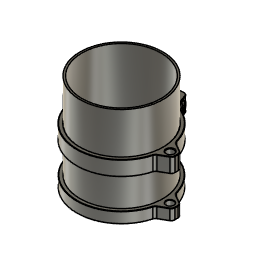
rear_44mm (Autodesk Fusion 360 design; units mm, degrees)
Autodesk Fusion 360 part; units mm, degrees
sketch "Sketch1" plane through (0, 0, 0) normal (0, 0, 1) x (1, 0, 0)
  circle A0 centre (0, 0) radius 22.2
  circle A1 centre (0, 0) radius 21.2
  dimension "d1" = 44.4
  dimension "d2" = 1
  constraint coincident A0.centre A1.centre
  measures "d1" diameter of A0
  measures "d2" distance of A0 A1
extrude "Extrude1" add sketch "Sketch1" along normal blind 50 makes body 1
ref_plane "WorkPlane1" through (0, 0, 20) normal (0, 0, 1) x (1, 0, 0)
sketch "Sketch2" plane through (0, 0, 20) normal (0, 0, 1) x (1, 0, 0)
  circle A0 centre (0, 0) radius 22.1
  circle A1 centre (0, 0) radius 24.1
  line L0 (0, 0) -> (0, 24.1) construction
  line L1 (-6.9118, 23.0876) -> (-4, 31.0876)
  line L2 (-4, 31.0876) -> (0, 31.0876)
  line L3 (0, 31.0876) -> (0, 24.1)
  line L4 (-6.9118, 23.0876) -> (0, 23.0876) construction
  line L5 (-4, 31.0876) -> (-4, 23.0876) construction
  line L6 (0, 0) -> (-0.3086, 22.0978)
  line L7 (-0.3086, 22.0978) -> (-0.3086, 31.0876)
  line L8 (6.9118, 23.0876) -> (4, 31.0876)
  line L9 (4, 31.0876) -> (0, 31.0876)
  line L10 (0.3086, 22.0978) -> (0.3086, 31.0876)
  line L11 (0, 0) -> (0.3086, 22.0978)
  circle A2 centre (-26.1, 0) radius 2
  line L12 (0, 0) -> (-24.1, 0) construction
  line L13 (-23.4467, 5.5733) -> (-29.6, 2.0207)
  line L14 (-29.6, 2.0207) -> (-29.6, 0)
  line L15 (-23.4467, -5.5733) -> (-29.6, -2.0207)
  line L16 (-29.6, -2.0207) -> (-29.6, 0)
  line L17 (23.4467, 5.5733) -> (29.6, 2.0207)
  line L18 (29.6, 2.0207) -> (29.6, 0)
  line L19 (29.6, -2.0207) -> (29.6, 0)
  line L20 (23.4467, -5.5733) -> (29.6, -2.0207)
  circle A3 centre (26.1, 0) radius 2
  dimension "d6" = 44.2
  dimension "d7" = 2
  dimension "d8" = 8
  dimension "d9" = 20
  dimension "d10" = 4
  dimension "d11" = 0.8
  dimension "d14" = 4
  dimension "d16" = 3.5
  dimension "d17" = 3.5
  dimension "d18" = 120
  constraint coincident A0.centre A1.centre
  constraint coincident A1 L0.end
  constraint vertical L0
  constraint coincident A1 L1.start
  constraint horizontal L2
  constraint perpendicular L2 L3
  constraint coincident L0 L4.end
  constraint horizontal L4
  constraint coincident L4 L5.end
  constraint perpendicular L4 L5
  constraint coincident A0 L6.end
  constraint coincident L2 L7.end
  constraint perpendicular L2 L7
  constraint symmetric L0 L1.start L8.start
  constraint symmetric L0 L1.end L8.end
  constraint symmetric L0 L2.end L3.start
  constraint symmetric L0 A0.centre A1.centre
  constraint symmetric L0 L6.end L10.start
  constraint symmetric L0 L7.end L10.end
  constraint coincident A1 L12.end
  constraint horizontal L12
  constraint coincident A2.centre L12
  constraint coincident A1 L13.start
  constraint vertical L14
  constraint tangent A1 A2
  constraint coincident L12 L14.end
  constraint symmetric L12 L13.start L15.start
  constraint symmetric L12 L13.end L15.end
  constraint symmetric L12 L14.end L16.end
  constraint symmetric L0 A2 A3
  constraint symmetric L0 L13.start L17.start
  constraint symmetric L0 L13.end L17.end
  constraint symmetric L0 L14.end L18.end
  constraint symmetric L0 L15.start L20.start
  constraint symmetric L0 L15.end L19.start
  measures "d6" diameter of A0
  measures "d7" distance of A0 A1
  measures "d8" distance of L2 L4
  measures "d9" angle of L1 L5
  measures "d10" distance of L1.end L3
  measures "d11" angle of L0 L6
  measures "d14" diameter of A2
  measures "d16" distance of A2.centre L14
  measures "d17" distance of A2.centre L13
  measures "d18" angle of L13 L14
extrude "Extrude2" add sketch "Sketch2" along normal blind 8 separate body contours A0 A1 L7 L10 | A1 L8 L9 L10 | A1 L1 L2 L7 | A1 L17 L18 L19 L20 | A1 L13 L14 L15 L16 picked at (22.6631, -1.702) makes body 2
sketch "Sketch3" plane through (-0.3086, 0, 0) normal (1, 0, 0) x (0, 1, 0)
  line L0 (22.0978, 20) -> (31.0876, 20)
  line L1 (31.0876, 20) -> (31.0876, 28)
  line L2 (31.0876, 28) -> (22.0978, 28)
  line L3 (22.0978, 28) -> (22.0978, 20)
  line L4 (22.0978, 24) -> (31.0876, 24) construction
  line L5 (26.5927, 28) -> (26.5927, 20) construction
  circle A0 centre (27.0876, 24) radius 1.4
  dimension "d19" = 2.8
  dimension "d20" = 4
  constraint midpoint L3 L4.start
  constraint midpoint L1 L4.end
  constraint midpoint L2 L5.start
  constraint perpendicular L2 L5
  constraint coincident L4 A0.centre
  measures "d19" diameter of A0
  measures "d20" distance of L1 A0.centre
extrude "Extrude3" cut sketch "Sketch3" along normal through all and the other way through all contours A0 bodies 2
sketch "Sketch4" plane through (0, 0, 28) normal (0, 0, 1) x (-1, 0, 0)
  circle A0 centre (-26.1, 0) radius 2
  circle A1 centre (26.1, 0) radius 2
  arc A2 (23.4467, 5.5733) -> (-23.4467, 5.5733) centre (0, 0) ccw
  line L0 (-23.4467, 5.5733) -> (-29.6, 2.0207)
  line L1 (-29.6, 2.0207) -> (-29.6, -2.0207)
  line L2 (-29.6, -2.0207) -> (-23.4467, -5.5733)
  arc A3 (-23.4467, -5.5733) -> (-6.9118, -23.0876) centre (0, 0) ccw
  line L3 (-6.9118, -23.0876) -> (-4, -31.0876)
  line L4 (-4, -31.0876) -> (-0.3086, -31.0876)
  line L5 (-0.3086, -31.0876) -> (-0.3086, -22.0978)
  arc A4 (0.3086, -22.0978) -> (-0.3086, -22.0978) centre (0, 0) ccw
  line L6 (0.3086, -22.0978) -> (0.3086, -31.0876)
  line L7 (0.3086, -31.0876) -> (4, -31.0876)
  line L8 (4, -31.0876) -> (6.9118, -23.0876)
  arc A5 (6.9118, -23.0876) -> (23.4467, -5.5733) centre (0, 0) ccw
  line L9 (23.4467, -5.5733) -> (29.6, -2.0207)
  line L10 (29.6, -2.0207) -> (29.6, 2.0207)
  line L11 (29.6, 2.0207) -> (23.4467, 5.5733)
  line L12 (-4, -31.0876) -> (-4, -21.735) construction
  constraint coincident L3.end L4.start
  constraint coincident A4 L12.end
  constraint perpendicular L4 L12
sketch "Sketch5" plane through (0, 0, 20) normal (0, 0, -1) x (1, 0, 0)
  circle A0 centre (26.1, 0) radius 2
  circle A1 centre (-26.1, 0) radius 2
  arc A2 (23.4467, 5.5733) -> (-23.4467, 5.5733) centre (0, 0) ccw
  line L0 (-23.4467, 5.5733) -> (-29.6, 2.0207)
  line L1 (-29.6, 2.0207) -> (-29.6, -2.0207)
  line L2 (-29.6, -2.0207) -> (-23.4467, -5.5733)
  arc A3 (-23.4467, -5.5733) -> (-6.9118, -23.0876) centre (0, 0) ccw
  line L3 (-6.9118, -23.0876) -> (-4, -31.0876)
  line L4 (-4, -31.0876) -> (-0.3086, -31.0876)
  line L5 (-0.3086, -31.0876) -> (-0.3086, -22.0978)
  arc A4 (0.3086, -22.0978) -> (-0.3086, -22.0978) centre (0, 0) ccw
  line L6 (0.3086, -22.0978) -> (0.3086, -31.0876)
  line L7 (0.3086, -31.0876) -> (4, -31.0876)
  line L8 (4, -31.0876) -> (6.9118, -23.0876)
  arc A5 (6.9118, -23.0876) -> (23.4467, -5.5733) centre (0, 0) ccw
  line L9 (23.4467, -5.5733) -> (29.6, -2.0207)
  line L10 (29.6, -2.0207) -> (29.6, 2.0207)
  line L11 (29.6, 2.0207) -> (23.4467, 5.5733)
  line L12 (4, -31.0876) -> (4, -21.735) construction
ref_plane "WorkPlane2" through (4, 31.0876, 28) normal (-1, 0, 0) x (0, -1, 0)
sketch "Sketch6" plane through (4, 0, 0) normal (-1, 0, 0) x (0, -1, 0)
  circle A0 centre (-27.0876, 24) radius 1.4
  circle A1 centre (-27.0876, 24) radius 1.4
  circle A2 centre (-27.0876, 24) radius 3
  dimension "d23" = 6
  constraint concentric A0 A2
  measures "d23" diameter of A2
extrude "Extrude4" cut sketch "Sketch6" against normal through all bodies 2
sketch "Sketch7" plane through (0.3086, 0, 0) normal (-1, 0, 0) x (0, -1, 0)
  circle A0 centre (-27.0876, 24) radius 1.4
  line L0 (-31.0876, 20) -> (-22.0978, 20)
  line L1 (-22.0978, 20) -> (-22.0978, 28)
  line L2 (-22.0978, 28) -> (-31.0876, 28)
  line L3 (-31.0876, 28) -> (-31.0876, 20)
  circle A1 centre (-27.0876, 24) radius 1.7
  dimension "d28" = 3.4
  constraint concentric A0 A1
  measures "d28" diameter of A1
extrude "Extrude6" cut sketch "Sketch7" against normal up to surface (3.6914 mm away) contours A1 bodies 2
fillet "Fillet1" radius 2 12 edges at (-29.6, -2.0207, 24) (-23.4467, -5.5733, 24) (-29.6, 2.0207, 24) (-23.4467, 5.5733, 24) (23.4467, -5.5733, 24) (29.6, -2.0207, 24) (29.6, 2.0207, 24) (23.4467, 5.5733, 24) (6.9118, 23.0876, 24) (-6.9118, 23.0876, 24) (4, 31.0876, 24) (-4, 31.0876, 24) on bodies 2
fillet "Fillet2" radius 0.5 4 edges at (0.3086, 31.0876, 24) (-0.3086, 31.0876, 24) (0.3086, 22.0978, 24) (-0.3086, 22.0978, 24) on bodies 2
chamfer "Chamfer1" distance 0.2 angle 45 4 edges at (4, 28.6726, 23.3853) (0.3086, 28.6726, 24.6147) (-0.3086, 25.7823, 24.5063) (-5.9654, 25.6876, 24) on bodies 2
fillet "Fillet5" radius 0.2 3 edges at (4, 29.8846, 22.9152) (6.5478, 24.0876, 24) (4.3316, 30.0876, 24) on bodies 2
chamfer "Chamfer2" distance 0.2 angle 45 32 edges at (-23.5921, 5.6629, 28) (-17.5696, 16.496, 28) (-7.0555, 23.2645, 28) (-5.5278, 26.8899, 28) (-3.7467, 30.7259, 28) (-1.7041, 31.0876, 28) (-0.455, 30.9412, 28) (-0.3086, 26.5866, 28) (-0.4487, 22.2384, 28) (0, -22.1, 28) (0.4487, 22.2384, 28) (0.3086, 26.5866, 28) (0.455, 30.9412, 28) (1.7041, 31.0876, 28) (3.7467, 30.7259, 28) (5.5278, 26.8899, 28) (7.0555, 23.2645, 28) (17.5696, 16.496, 28) (23.5921, 5.6629, 28) (26.3878, 3.8753, 28) (29.3321, 1.866, 28) (29.6, 0, 28) (29.3321, -1.866, 28) (26.3878, -3.8753, 28) (23.5921, -5.6629, 28) (0, -24.1, 28) (-23.5921, -5.6629, 28) (-26.3878, -3.8753, 28) (-29.3321, -1.866, 28) (-29.6, 0, 28) (-29.3321, 1.866, 28) (-26.3878, 3.8753, 28) on bodies 2
chamfer "Chamfer3" distance 0.3 angle 45 36 edges at (-27.9647, 0.7232, 28) (24.2353, 0.7232, 28) (26.3878, 3.8753, 20) (29.3321, 1.866, 20) (29.6, 0, 20) (29.3321, -1.866, 20) (26.3878, -3.8753, 20) (23.5921, -5.6629, 20) (0, -24.1, 20) (-23.5921, -5.6629, 20) (-26.3878, -3.8753, 20) (-29.3321, -1.866, 20) (-29.6, 0, 20) (-29.3321, 1.866, 20) (-26.3878, 3.8753, 20) (-23.5921, 5.6629, 20) (-17.5696, 16.496, 20) (-7.0555, 23.2645, 20) (-5.5278, 26.8899, 20) (-3.7467, 30.7259, 20) (-1.7041, 31.0876, 20) (-0.455, 30.9412, 20) (-0.3086, 26.5866, 20) (-0.4487, 22.2384, 20) (0, -22.1, 20) (0.4487, 22.2384, 20) (0.3086, 26.5866, 20) (0.455, 30.9412, 20) (1.7041, 31.0876, 20) (3.7467, 30.7259, 20) (5.5278, 26.8899, 20) (7.0555, 23.2645, 20) (17.5696, 16.496, 20) (23.5921, 5.6629, 20) (24.2353, 0.7232, 20) (-27.9647, 0.7232, 20) on bodies 2
sketch "Sketch8" plane through (0, 0, 0) normal (0, 0, 1) x (1, 0, 0)
  circle A0 centre (0, 0) radius 22
  circle A1 centre (0, 0) radius 24
  line L0 (23.3435, 5.5752) -> (29.5, 2.0207)
  line L1 (29.5, 2.0207) -> (29.5, 0)
  line L2 (0, 0) -> (24, 0) construction
  line L3 (23.3435, -5.5752) -> (29.5, -2.0207)
  line L4 (29.5, -2.0207) -> (29.5, 0)
  line L5 (0, 0) -> (0, 22) construction
  line L6 (-23.3435, 5.5752) -> (-29.5, 2.0207)
  line L7 (-29.5, 2.0207) -> (-29.5, 0)
  line L8 (-29.5, -2.0207) -> (-29.5, 0)
  line L9 (-23.3435, -5.5752) -> (-29.5, -2.0207)
  circle A2 centre (26, 0) radius 2
  circle A3 centre (-26, 0) radius 2
  line L10 (0, 0) -> (-26, 0) construction
  dimension "d38" = 44
  dimension "d39" = 2
  dimension "d41" = 3.5
  dimension "d42" = 3.5
  dimension "d43" = 120
  dimension "d46" = 4
  dimension "d47" = 4
  constraint coincident A0.centre A1.centre
  constraint coincident A1 L0.start
  constraint vertical L1
  constraint coincident A1 L2.end
  constraint horizontal L2
  constraint symmetric L0.start L2 L3.start
  constraint symmetric L0.end L2 L3.end
  constraint symmetric L1.end L2 L4.end
  constraint coincident A0 L5.end
  constraint perpendicular L2 L5
  constraint symmetric L0.start L5 L6.start
  constraint symmetric L0.end L5 L6.end
  constraint symmetric L1.end L5 L7.end
  constraint symmetric L3.start L5 L9.start
  constraint symmetric L3.end L5 L8.start
  constraint tangent A1 A2
  constraint coincident L2 A2.centre
  constraint tangent A1 A3
  constraint coincident A3.centre L10.end
  constraint horizontal L10
  measures "d38" diameter of A0
  measures "d39" distance of A0 A1
  measures "d41" distance of L0 A2.centre
  measures "d42" distance of L1 A2.centre
  measures "d43" angle of L0 L1
  measures "d46" diameter of A2
  measures "d47" diameter of A3
extrude "Extrude7" add sketch "Sketch8" along normal blind 4 separate body makes body 3
extrude "Extrude8" add sketch "Sketch8" against normal blind 2 contours A0 | A1 | A1 L0 L1 L3 L4 | A1 L6 L7 L8 L9 bodies 3
fillet "Fillet3" radius 2 8 edges at (23.3435, -5.5752, 1) (29.5, -2.0207, 1) (29.5, 2.0207, 1) (23.3435, 5.5752, 1) (-23.3435, 5.5752, 1) (-29.5, 2.0207, 1) (-29.5, -2.0207, 1) (-23.3435, -5.5752, 1) on bodies 3
chamfer "Chamfer4" distance 0.2 angle 45 19 edges at (-29.2321, -1.866, 4) (-29.5, 0, 4) (-29.2321, 1.866, 4) (-26.2856, 3.8765, 4) (-23.4884, 5.6646, 4) (0, 24, 4) (23.4884, 5.6646, 4) (26.2856, 3.8765, 4) (29.2321, 1.866, 4) (29.5, 0, 4) (29.2321, -1.866, 4) (26.2856, -3.8765, 4) (23.4884, -5.6646, 4) (0, -24, 4) (-23.4884, -5.6646, 4) (-26.2856, -3.8765, 4) (-27.8647, 0.7232, 4) (-20.5112, 7.9555, 4) (24.1353, 0.7232, 4) on bodies 3
chamfer "Chamfer5" distance 0.3 angle 45 18 edges at (26.2856, -3.8765, -2) (23.4884, -5.6646, -2) (0, -24, -2) (-23.4884, -5.6646, -2) (-26.2856, -3.8765, -2) (-29.2321, -1.866, -2) (-29.5, 0, -2) (-29.2321, 1.866, -2) (-26.2856, 3.8765, -2) (-23.4884, 5.6646, -2) (0, 24, -2) (23.4884, 5.6646, -2) (26.2856, 3.8765, -2) (29.2321, 1.866, -2) (29.5, 0, -2) (29.2321, -1.866, -2) (-27.8647, -0.7232, -2) (24.1353, -0.7232, -2) on bodies 3
fillet "Fillet4" radius 0.2 1 edges at (-20.5112, 7.9555, 0) on bodies 3
equation "d11 = ( 1.6 / 2 ) * 1 deg"
named bodies: "mocked_scope_44mm", "scope_collar_44mm", "scope_cap_44mm"
